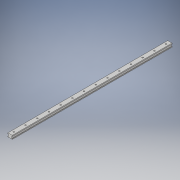
# Autodesk Inventor part: Rail
Saved by Autodesk Inventor 2017 (Build 210142000, 142)
## iProperties
Created: 2017-05-03
Part Number: Rail
Material: Generic
Document SubType Name: Modeling
Designer: Jon
Density: 1 g/cm^3
Appearance: Default
Author: Jon
Autodesk Inventor part; units mm, degrees
ref_plane "YZ Plane" through (0, 0, 0) normal (1, 0, 0) x (0, 1, 0)
ref_plane "XZ Plane" through (0, 0, 0) normal (0, 1, 0) x (-1, 0, 0)
ref_plane "XY Plane" through (0, 0, 0) normal (0, 0, 1) x (1, 0, 0)
sketch "Sketch1" plane through (0, 0, 0) normal (0, 1, 0) x (-1, 0, 0)
  point P0 (0, 0)
sketch "Sketch2" plane through (0, 0, 0) normal (0, 0, 1) x (1, 0, 0)
  line L0 (-10.9925, 4.7492) -> (9.0481, 4.7492)
  line L1 (9.0481, -11.7227) -> (-10.9925, -11.7227)
  line L2 (7.0415, 0.5074) -> (7.0415, -8.7636)
  line L3 (-8.9986, -8.7636) -> (-8.9986, 0.5074)
  line L4 (-8.9986, 0.5074) -> (-10.9925, 0.5074)
  line L5 (-8.9986, -8.7636) -> (-10.9925, -8.7636)
  line L6 (7.0415, -8.7636) -> (9.0481, -8.7636)
  line L7 (7.0415, 0.5074) -> (9.0481, 0.5074)
  line L8 (9.0481, 4.7492) -> (9.0481, 0.5074)
  line L9 (9.0481, -8.7636) -> (9.0481, -11.7227)
  line L10 (-10.9925, -11.7227) -> (-10.9925, -8.7636)
  line L11 (-10.9925, 0.5074) -> (-10.9925, 4.7492)
  point P0 (0, 0)
  constraints: 24 end point, 8 perpendicular, 6 parallel, 2 horizontal
extrude "Extrusion1" add sketch "Sketch2" along normal blind 737.362
sketch "Sketch3" plane through (-10.9925, 4.7492, 0) normal (0, 1, 0) x (1, 0, 0)
  circle A0 centre (10.0203, -179.451) radius 2.8956
  line L0 (0, 0) -> (20.0406, 0) projected
  circle A1 centre (10.0203, -233.5403) radius 2.8956
  line L1 (20.0406, 0) -> (20.0406, -737.362) projected
  line L2 (0, 0) -> (0, -737.362) projected
  circle A2 centre (10.0203, -287.6296) radius 2.8956
  circle A3 centre (10.0203, -341.7189) radius 2.8956
  circle A4 centre (10.0203, -395.8082) radius 2.8956
  circle A5 centre (10.0203, -449.8975) radius 2.8956
  circle A6 centre (10.0203, -503.9868) radius 2.8956
  circle A7 centre (10.0203, -558.0761) radius 2.8956
  circle A8 centre (10.0203, -612.1654) radius 2.8956
  circle A9 centre (10.0203, -666.2547) radius 2.8956
  circle A10 centre (10.0203, -720.344) radius 2.8956
  line L3 (20.0406, -737.362) -> (0, -737.362) projected
  circle A11 centre (10.0203, -125.3617) radius 2.8956
  circle A12 centre (10.0203, -71.2724) radius 2.8956
  circle A13 centre (10.0203, -17.1831) radius 2.8956
  point P0 (10.9925, 0)
  dimension "d16" = 20.0406
  dimension "d17" = 54.0893
  dimension "d19" = 54.0893
  dimension "d20" = 54.0893
  dimension "d21" = 54.0893
  dimension "d22" = 54.0893
  dimension "d23" = 54.0893
  dimension "d24" = 54.0893
  dimension "d25" = 54.0893
  dimension "d26" = 54.0893
  dimension "d27" = 54.0893
  dimension "d28" = 17.018
  dimension "d29" = 54.0893
  dimension "d30" = 54.0893
  dimension "d31" = 54.0893
  dimension "d33" = 10.0203
  dimension "d34" = 10.0203
  dimension "d35" = 10.0203
  dimension "d36" = 10.0203
  dimension "d37" = 10.0203
  constraints: 14 centre point
  measures "d16" distance of L0.start L0.end
  measures "d17" distance of A1.centre A0.centre
  measures "d19" distance of A2.centre A1.centre
  measures "d20" distance of A2.centre A3.centre
  measures "d21" distance of A3.centre A4.centre
  measures "d22" distance of A4.centre A5.centre
  measures "d23" distance of A5.centre A6.centre
  measures "d24" distance of A6.centre A7.centre
  measures "d25" distance of A7.centre A8.centre
  measures "d26" distance of A8.centre A9.centre
  measures "d27" distance of A9.centre A10.centre
  measures "d28" distance from line of L3 A10.centre
  measures "d29" distance of A0.centre A11.centre
  measures "d30" distance of A11.centre A12.centre
  measures "d31" distance of A13.centre A12.centre
  measures "d33" distance from line of L2 A13.centre
  measures "d34" distance from line of L1 A13.centre
  measures "d35" distance from line of L2 A12.centre
  measures "d36" distance from line of L2 A11.centre
  measures "d37" distance from line of L2 A10.centre
hole "Hole1" at (-0.9722, 4.7492, 17.1831) at (-0.9722, 4.7492, 71.2724) at (-0.9722, 4.7492, 125.3617) at (-0.9722, 4.7492, 179.451) at (-0.9722, 4.7492, 233.5403) at (-0.9722, 4.7492, 287.6296) at (-0.9722, 4.7492, 341.7189) at (-0.9722, 4.7492, 395.8082) at (-0.9722, 4.7492, 449.8975) at (-0.9722, 4.7492, 503.9868) at (-0.9722, 4.7492, 558.0761) at (-0.9722, 4.7492, 612.1654) at (-0.9722, 4.7492, 666.2547) at (-0.9722, 4.7492, 720.344) direction (0, -1, 0) diameter 5.969 end through all
sketch "Sketch4" plane through (-10.9925, 4.7492, 0) normal (0, 1, 0) x (1, 0, 0)
  point P0 (10.9925, 0)
sketch "Sketch5" plane through (-10.9925, -11.7227, 0) normal (0, -1, 0) x (1, 0, 0)
  point P0 (10.9925, 0)
sketch "Sketch6" plane through (-10.9925, -11.7227, 0) normal (0, -1, 0) x (1, 0, 0)
  line L0 (20.0406, 0) -> (20.0406, 737.362) projected
  line L1 (20.0406, 0) -> (0, 0) projected
  circle A0 centre (10.0203, 666.2547) radius 2.9845 projected
  line L2 (0, 737.362) -> (20.0406, 737.362) projected
  line L3 (0, 0) -> (0, 737.362) projected
  point P0 (10.9925, 0)
  point P1 (10.0203, 125.222)
  point P2 (10.0203, 179.324)
  point P3 (10.0203, 233.426)
  point P4 (10.0203, 287.528)
  point P5 (10.0203, 341.63)
  point P6 (10.0203, 395.732)
  point P7 (10.0203, 449.834)
  point P8 (10.0203, 503.936)
  point P9 (10.0203, 558.038)
  point P10 (10.0203, 612.14)
  point P11 (10.0203, 720.344)
  point P12 (10.0203, 666.242)
  point P13 (10.0203, 71.12)
  point P14 (10.0203, 17.018)
  dimension "d59" = 10.0203
  dimension "d60" = 10.0203
  dimension "d61" = 54.102
  dimension "d62" = 54.102
  dimension "d63" = 10.0203
  dimension "d64" = 54.102
  dimension "d65" = 10.0203
  dimension "d66" = 54.102
  dimension "d67" = 54.102
  dimension "d68" = 54.102
  dimension "d69" = 54.102
  dimension "d70" = 54.102
  dimension "d71" = 54.102
  dimension "d74" = 54.102
  dimension "d75" = 54.102
  dimension "d76" = 17.018
  dimension "d77" = 10.0203
  dimension "d78" = 10.0203
  dimension "d79" = 10.0203
  dimension "d80" = 10.0203
  dimension "d81" = 10.0203
  dimension "d82" = 54.102
  dimension "d83" = 54.102
  dimension "d84" = 10.0203
  dimension "d85" = 10.0203
  dimension "d86" = 10.0203
  measures "d59" distance from line of L0 point (10.02, 125.222)
  measures "d60" distance from line of L0 point (10.02, 179.324)
  measures "d61" distance of point (10.02, 125.222) point (10.02, 179.324)
  measures "d62" distance of point (10.02, 179.324) point (10.02, 233.426)
  measures "d63" distance from line of L0 point (10.02, 233.426)
  measures "d64" distance of point (10.02, 287.528) point (10.02, 233.426)
  measures "d65" distance from line of L0 point (10.02, 287.528)
  measures "d66" distance of point (10.02, 287.528) point (10.02, 341.63)
  measures "d67" distance of point (10.02, 341.63) point (10.02, 395.732)
  measures "d68" distance of point (10.02, 395.732) point (10.02, 449.834)
  measures "d69" distance of point (10.02, 503.936) point (10.02, 449.834)
  measures "d70" distance of point (10.02, 558.038) point (10.02, 503.936)
  measures "d71" distance of point (10.02, 612.14) point (10.02, 558.038)
  measures "d74" distance of point (10.02, 666.242) point (10.02, 612.14)
  measures "d75" distance of point (10.02, 666.242) point (10.02, 720.344)
  measures "d76" distance from line of L2 point (10.02, 720.344)
  measures "d77" distance from line of L3 point (10.02, 720.344)
  measures "d78" distance from line of L0 point (10.02, 720.344)
  measures "d79" distance from line of L3 point (10.02, 666.242)
  measures "d80" distance from line of L3 point (10.02, 612.14)
  measures "d81" distance from line of L3 point (10.02, 558.038)
  measures "d82" distance of point (10.02, 71.12) point (10.02, 125.222)
  measures "d83" distance of point (10.02, 71.12) point (10.02, 17.018)
  measures "d84" distance from line of L0 point (10.02, 17.018)
  measures "d85" distance from line of L0 point (10.02, 71.12)
  measures "d86" distance from line of L3 point (10.02, 503.936)
sketch "Sketch7" plane through (-10.9925, -11.7227, 0) normal (0, -1, 0) x (1, 0, 0)
  point P0 (10.9925, 0)
equation "\"d19\" = d17"
equation "\"d20\" = d17"
equation "\"d21\" = d17"
equation "\"d22\" = d17"
equation "\"d23\" = d17"
equation "\"d24\" = d17"
equation "\"d25\" = d17"
equation "\"d26\" = d17"
equation "\"d27\" = d17"
equation "\"d29\" = d17"
equation "\"d30\" = d17"
equation "\"d31\" = d17"
equation "\"d61\" = d50"
equation "\"d62\" = d50"
equation "\"d64\" = d50"
equation "\"d66\" = d50"
equation "\"d67\" = d50"
equation "\"d68\" = d50"
equation "\"d69\" = d50"
equation "\"d70\" = d50"
equation "\"d71\" = d50"
equation "\"d74\" = d50"
equation "\"d75\" = d50"
equation "\"d79\" = d77"
equation "\"d80\" = d77"
equation "\"d81\" = d77"
equation "\"d82\" = d61"
equation "\"d83\" = d82"
equation "\"d86\" = d77"
equation "\"d50\" = 54.102"
body "Solid1"
